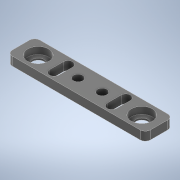
# Autodesk Inventor part: Rack support b
Saved by Autodesk Inventor 2022 (Build 260153000, 153)
## iProperties
Created: 2022-03-06
Part Number: Rack support b
Material: Genérico
Document SubType Name: Modeling
Designer: JK
Density: 1 g/cm^3
Appearance: Suave - Negro
Author: JK
Autodesk Inventor part; units mm, degrees
ref_plane "YZ Plane" through (0, 0, 0) normal (1, 0, 0) x (0, 1, 0)
ref_plane "XZ Plane" through (0, 0, 0) normal (0, 1, 0) x (-1, 0, 0)
ref_plane "XY Plane" through (0, 0, 0) normal (0, 0, 1) x (1, 0, 0)
sketch "Boceto1" plane through (0, 0, 0) normal (0, 1, 0) x (-1, 0, 0)
  line L0 (-40, 8) -> (40, 8)
  line L1 (40, 8) -> (40, -8)
  line L2 (40, -8) -> (-40, -8)
  line L3 (-40, -8) -> (-40, 8)
  line L4 (-40, 8) -> (40, -8) construction
  line L5 (40, 8) -> (-40, -8) construction
  circle A0 centre (-16.7, 4) radius 2.7
  circle A1 centre (-16.7, -4) radius 2.7
  circle A2 centre (16.7, 4) radius 2.7
  circle A3 centre (16.7, -4) radius 2.7
  line L6 (19.4, 4) -> (14, 4)
  line L7 (14, 4) -> (14, -4)
  line L8 (14, -4) -> (19.4, -4)
  line L9 (19.4, -4) -> (19.4, 4)
  line L10 (-14, 4) -> (-19.4, 4)
  line L11 (-19.4, 4) -> (-19.4, -4)
  line L12 (-19.4, -4) -> (-14, -4)
  line L13 (-14, -4) -> (-14, 4)
  point P0 (0, 0)
  point P1 (16.7, -4)
  point P2 (16.7, 4)
  point P3 (-16.7, -4)
  point P4 (-16.7, 4)
  point P5 (19.4, -4)
  point P6 (-14, -4)
  point P7 (-19.4, -4)
  point P8 (-19.4, 4)
  dimension "d2" = 5.4
  dimension "d0" = 80
  dimension "d1" = 16
  dimension "d3" = 4
  dimension "d4" = 8
  dimension "d5" = 23.3
  dimension "d35" = 23.3
  constraints: 28 end point, 7 midpoint, 6 parallel, 3 horizontal, 3 perpendicular, 3 vertical, 2 horizontal alignment, 1 centre point, 1 point on line, 1 tangent, 1 vertical alignment, 11 other
  measures "d0" distance of L1.end L2.end
  measures "d1" distance of L0.end L1.end
  measures "d3" vertical distance of point (0, 0) point (-16.7, 4)
  measures "d4" distance of L10.end L11.end
  measures "d5" distance from line of L3 point (-16.7, 4)
  measures "d35" distance from line of L1 point (16.7, -4)
extrude "Extrusión1" add sketch "Boceto1" along normal blind 5
fillet "Empalme2" radius 3 4 edges at (-40, 2.5, 8) (-40, 2.5, -8) (40, 2.5, 8) (40, 2.5, -8)
sketch "Boceto6" plane through (0, 5, 0) normal (0, 1, 0) x (1, 0, 0)
  circle A0 centre (-30, 0) radius 6.125
  circle A1 centre (30, 0) radius 6.125
  point P0 (0, 0)
  dimension "d27" = 12.25
  dimension "d28" = 30
  dimension "d29" = 30
  constraints: 2 centre point, 1 equal radius
  measures "d27" diameter of A0
  measures "d28" distance of point (0, 0) A1.centre
  measures "d29" distance of A0.centre point (0, 0)
extrude "Extrusión6" cut sketch "Boceto6" against normal through all
sketch "Boceto7" plane through (0, 0, 0) normal (0, -1, 0) x (1, 0, 0)
  circle A0 centre (-30, 0) radius 6.125 projected
  circle A1 centre (30, 0) radius 6.125 projected
  circle A2 centre (-30, 0) radius 3.5
  circle A3 centre (30, 0) radius 3.5
  point P0 (0, 0)
  point P1 (18.5632, -5.9541)
  point P2 (18.5632, 5.9541)
  dimension "d32" = 7
  constraints: 2 centre point, 2 coincident, 1 equal radius, 1 other
  measures "d32" diameter of A2
extrude "Extrusión7" add sketch "Boceto7" against normal blind 1
sketch "Boceto9" plane through (0, 5, 0) normal (0, 1, 0) x (1, 0, 0)
  circle A0 centre (-7, 0.0746) radius 2.7
  circle A1 centre (7, 0.0746) radius 2.7
  point P0 (0, 0)
  dimension "d36" = 5.4
  dimension "d39" = 7
  dimension "d40" = 7
  constraints: 2 centre point, 1 coincident, 1 equal radius, 1 other
  measures "d36" diameter of A0
  measures "d39" horizontal distance of point (-7, 0.075) point (0, 0)
  measures "d40" horizontal distance of point (0, 0) A1.centre
extrude "Extrusión8" cut sketch "Boceto9" against normal through all
sketch "Boceto5" plane through (0, 0, 0) normal (0, -1, 0) x (1, 0, 0)
  circle A0 centre (-30, -4.1) radius 1.7 projected
  circle A1 centre (-30, -4.1) radius 2.875
  circle A2 centre (20, -4.1) radius 1.7 projected
  circle A3 centre (20, -4.1) radius 2.875
  line L0 (-33.3198, -4.1) -> (-31.6599, -1.225)
  line L1 (-31.6599, -1.225) -> (-28.3401, -1.225)
  line L2 (-28.3401, -1.225) -> (-26.6802, -4.1)
  line L3 (-26.6802, -4.1) -> (-28.3401, -6.975)
  line L4 (-28.3401, -6.975) -> (-31.6599, -6.975)
  line L5 (-31.6599, -6.975) -> (-33.3198, -4.1)
  line L6 (16.6802, -4.1) -> (18.3401, -1.225)
  line L7 (18.3401, -1.225) -> (21.6599, -1.225)
  line L8 (21.6599, -1.225) -> (23.3198, -4.1)
  line L9 (23.3198, -4.1) -> (21.6599, -6.975)
  line L10 (21.6599, -6.975) -> (18.3401, -6.975)
  line L11 (18.3401, -6.975) -> (16.6802, -4.1)
  point P0 (0, 0)
  dimension "d24" = 5.75
  constraints: 24 end point, 4 coincident, 2 centre point, 2 tangent, 1 equal radius, 1 horizontal, 1 horizontal alignment, 26 other
  measures "d24" diameter of A1
